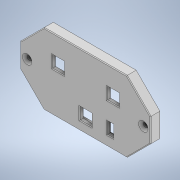
# Autodesk Inventor part: ideal_diode_enclosure
Saved by Autodesk Inventor 2021 (Build 250183000, 183)
## iProperties
Created: 2021-01-31
Part Number: ideal_diode_enclosure
Material: Generic
Document SubType Name: Modeling
Designer: oskar
Density: 1 g/cm^3
Appearance: Default
Author: oskar
## iProperties of the stored document _3DPrint.ipt
Created: 2021-01-31
Part Number: _3DPrint
Material: Generic
Document SubType Name: Modeling
Designer: oskar
Density: 1 g/cm^3
Appearance: Default
Author: oskar
Autodesk Inventor part; units mm, degrees
ref_plane "YZ Plane" through (0, 0, 0) normal (1, 0, 0) x (0, 1, 0)
ref_plane "XZ Plane" through (0, 0, 0) normal (0, 1, 0) x (-1, 0, 0)
ref_plane "XY Plane" through (0, 0, 0) normal (0, 0, 1) x (1, 0, 0)
sketch "Sketch1" plane through (0, 0, 0) normal (0, 0, 1) x (1, 0, 0)
  line L0 (-28, 3.75) -> (-18, 3.75)
  line L1 (-18, 3.75) -> (-18, 13.75)
  line L2 (-18, 13.75) -> (-28, 13.75)
  line L3 (-28, 13.75) -> (-28, 3.75)
  line L4 (-28, 3.75) -> (-18, 13.75) construction
  line L5 (-18, 3.75) -> (-28, 13.75) construction
  line L6 (18.38, 3.75) -> (28.38, 3.75)
  line L7 (28.38, 3.75) -> (28.38, 13.75)
  line L8 (28.38, 13.75) -> (18.38, 13.75)
  line L9 (18.38, 13.75) -> (18.38, 3.75)
  line L10 (18.38, 3.75) -> (28.38, 13.75) construction
  line L11 (28.38, 3.75) -> (18.38, 13.75) construction
  line L12 (-4.75, -12.5) -> (5.25, -12.5)
  line L13 (5.25, -12.5) -> (5.25, -22.5)
  line L14 (5.25, -22.5) -> (-4.75, -22.5)
  line L15 (-4.75, -22.5) -> (-4.75, -12.5)
  line L16 (-4.75, -12.5) -> (5.25, -22.5) construction
  line L17 (5.25, -12.5) -> (-4.75, -22.5) construction
  circle A0 centre (-23, 8.75) radius 1.925 construction
  circle A1 centre (23.38, 8.75) radius 1.925 construction
  circle A2 centre (0.25, -17.5) radius 1.925 construction
  line L18 (21.5954, -14.7725) -> (21.5954, -18.3725) construction
  line L19 (19.9954, -14.7725) -> (21.5954, -14.7725) construction
  line L20 (19.9954, -18.3725) -> (19.9954, -14.7725) construction
  line L21 (21.5954, -18.3725) -> (19.9954, -18.3725) construction
  line L22 (21.5454, -18.3225) -> (20.0454, -18.3225) construction
  line L23 (20.0454, -18.3225) -> (20.0454, -16.8225) construction
  line L24 (20.0454, -16.8225) -> (21.5454, -16.8225) construction
  line L25 (21.5454, -16.8225) -> (21.5454, -18.3225) construction
  line L26 (18.4, -21.5) -> (23.4, -21.5)
  line L27 (23.4, -21.5) -> (23.4, -11.5)
  line L28 (23.4, -11.5) -> (18.4, -11.5)
  line L29 (18.4, -11.5) -> (18.4, -21.5)
  line L30 (18.4, -21.5) -> (23.4, -11.5) construction
  line L31 (23.4, -21.5) -> (18.4, -11.5) construction
  circle A3 centre (22.55, -16.5) radius 0.45 construction
  circle A4 centre (19.25, -16.5) radius 0.45 construction
  line L32 (19.25, -16.5) -> (22.55, -16.5) construction
  line L33 (-45, -30) -> (45, -30)
  line L34 (45, -30) -> (45, 30)
  line L35 (45, 30) -> (-45, 30)
  line L36 (-45, 30) -> (-45, -30)
  line L37 (-45, -30) -> (45, 30) construction
  line L38 (45, -30) -> (-45, 30) construction
  line L39 (-30, 25) -> (30, 25) projected
  line L40 (35, 20) -> (35, -20) projected
  point P0 (0, 0)
  point P1 (23.38, 8.75)
  point P2 (0.25, -17.5)
  point P3 (20.9, -16.5)
  point P4 (20.9, -16.5)
  dimension "d0" = 10
  dimension "d3" = 5
  dimension "d4" = 10
  dimension "d5" = 10
  dimension "d6" = 5
  constraints: 62 end point, 16 midpoint, 10 parallel, 6 horizontal, 5 equal length, 5 perpendicular, 3 coincident
  measures "d0" distance of L0.end L1.end
  measures "d3" distance of L28.end L27.end
  measures "d4" distance of L27.end L26.end
  measures "d5" distance between parallel lines of L40 L34
  measures "d6" distance between parallel lines of L35 L39
extrude "Extrusion1" add sketch "Sketch1" along normal blind 3
sketch "Sketch2" plane through (0, 0, 0) normal (0, 0, -1) x (-1, 0, 0)
  line L0 (36, 26) -> (-36, 26)
  line L1 (-36, 26) -> (-36, -26)
  line L2 (-36, -26) -> (36, -26)
  line L3 (36, -26) -> (36, 26)
  line L4 (36, 26) -> (-36, -26) construction
  line L5 (-36, 26) -> (36, -26) construction
  line L6 (-30, -25) -> (30, -25) projected
  line L7 (35, -20) -> (35, 20) projected
  line L8 (-45, -30) -> (-45, 30) projected
  line L9 (45, -30) -> (-45, -30) projected
  line L10 (45, 30) -> (45, -30) projected
  line L11 (-45, 30) -> (45, 30) projected
  line L12 (-18.4, -21.5) -> (-18.4, -11.5) projected
  line L13 (-23.4, -21.5) -> (-18.4, -21.5) projected
  line L14 (-23.4, -11.5) -> (-23.4, -21.5) projected
  line L15 (-18.4, -11.5) -> (-23.4, -11.5) projected
  line L16 (4.75, -12.5) -> (-5.25, -12.5) projected
  line L17 (4.75, -22.5) -> (4.75, -12.5) projected
  line L18 (-5.25, -22.5) -> (4.75, -22.5) projected
  line L19 (-5.25, -12.5) -> (-5.25, -22.5) projected
  line L20 (-18.38, 3.75) -> (-18.38, 13.75) projected
  line L21 (-28.38, 3.75) -> (-18.38, 3.75) projected
  line L22 (-28.38, 13.75) -> (-28.38, 3.75) projected
  line L23 (-18.38, 13.75) -> (-28.38, 13.75) projected
  line L24 (28, 3.75) -> (28, 13.75) projected
  line L25 (18, 3.75) -> (28, 3.75) projected
  line L26 (18, 13.75) -> (18, 3.75) projected
  line L27 (28, 13.75) -> (18, 13.75) projected
  point P0 (0, 0)
  dimension "d9" = 1
  dimension "d10" = 1
  constraints: 12 end point, 2 midpoint, 2 parallel, 1 horizontal, 1 perpendicular
  measures "d9" distance between parallel lines of L2 L6
  measures "d10" distance between parallel lines of L3 L7
extrude "Extrusion2" add sketch "Sketch2" along normal blind 5 contours L8 L11 L10 L9
chamfer "Chamfer1" distance 10 angle 45 4 edges at (-45, -30, -1) (45, -30, -1) (45, 30, -1) (-45, 30, -1)
sketch "Sketch3" plane through (0, 0, 3) normal (0, 0, 1) x (1, 0, 0)
  line L0 (45, -20) -> (45, 20) projected
  line L1 (45, -20) -> (55, -10)
  line L2 (55, -10) -> (55, 10)
  line L3 (55, 10) -> (45, 20)
  line L4 (45, -20) -> (35, -30) projected
  line L5 (35, 30) -> (45, 20) projected
  line L6 (-65, 0) -> (75, 0) construction
  point P0 (0, 0)
  point P1 (49, 0)
  dimension "d16" = 10
  dimension "d17" = 6
  constraints: 6 end point, 2 collinear, 1 parallel, 1 point on line
  measures "d16" horizontal distance of L2.end L0.end
  measures "d17" distance from line of L2 point (49, 0)
extrude "Extrusion3" add sketch "Sketch3" against normal up to surface (8 mm away)
hole "Hole1" at (49, 0, 3) direction (0, 0, -1) diameter 4 end through all countersink diameter 8 countersink angle 90
mirror "Mirror1" about plane through (0, 0, 0) normal (1, 0, 0) of "Extrusion3", "Hole1"
chamfer "Chamfer2" distance 0.6 angle 45 24 edges at (45, -20, 3) (55, 0, 3) (45, 20, 3) (0, 30, 3) (-45, 20, 3) (-55, 0, 3) (-45, -20, 3) (0, -30, 3) (-28, 8.75, 3) (-23, 3.75, 3) (-18, 8.75, 3) (-23, 13.75, 3) (23.38, 13.75, 3) (28.38, 8.75, 3) (23.38, 3.75, 3) (18.38, 8.75, 3) (20.9, -11.5, 3) (18.4, -16.5, 3) (20.9, -21.5, 3) (23.4, -16.5, 3) (5.25, -17.5, 3) (0.25, -22.5, 3) (-4.75, -17.5, 3) (0.25, -12.5, 3)
body "Solid1"
